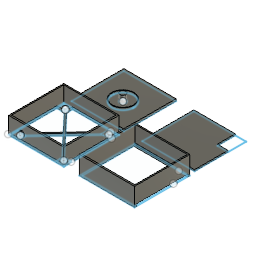
Enclosure_V2 (Autodesk Fusion 360 design; units mm, degrees)
part number: 2025-12-09-16-31-27-401
Autodesk Fusion 360 part; units mm, degrees
note: some values were not read from the file. Set by a fixed rule: which sketch regions a step uses.
sketch "Sketch1" plane through (0, 0, 0) normal (0, 0, 1) x (1, 0, 0)
  line L0 (19.5907, 74) -> (19.5907, 72.7904)
  line L1 (19.5907, 77.7937) -> (19.5907, 74)
  line L2 (78.8597, 77.7937) -> (71.7215, 77.7937)
  line L3 (44.546, 43.5668) -> (19.5907, 70.0195)
  line L4 (71.0242, 15.5) -> (46.0059, 42.0194)
  line L5 (78.8597, 70.2937) -> (78.8597, 77.7937)
  circle A0 centre (14.9411, 72.7904) radius 2.25
  circle A1 centre (73.9409, 72.7904) radius 2.25
  circle A2 centre (14.9411, 72.7904) radius 2.25
  line L6 (81.14, 79.55) -> (81.14, 4.55)
  line L7 (7.8597, 68.5) -> (7.8597, 77.7937)
  line L8 (71.0289, 68.5) -> (46.0059, 42.0194)
  line L9 (19.5907, 72.7904) -> (19.5907, 70.0195)
  circle A3 centre (14.9411, 72.7904) radius 2.25
  circle A4 centre (73.9409, 72.7904) radius 2.25
  line L10 (14, 68.5) -> (7.8597, 68.5)
  line L11 (18, 68.5) -> (14.9411, 68.5)
  line L12 (7.8597, 77.7937) -> (78.8597, 77.7937)
  line L13 (7.8597, 77.7937) -> (19.5907, 77.7937)
  line L14 (44.546, 43.5668) -> (68.0226, 68.411)
  line L15 (78.8597, 70.2937) -> (80.1709, 70.2937)
  line L16 (14, 68.5) -> (14.9411, 68.5)
  line L17 (6.14, 79.55) -> (81.14, 79.55)
  line L18 (6.14, 4.55) -> (6.14, 79.55)
  line L19 (7.8597, 6.7937) -> (7.8597, 77.7937)
  line L20 (78.8597, 77.7937) -> (78.8597, 6.7937)
  line L21 (78.8597, 15.5) -> (78.8597, 70.2937)
  line L22 (18, 68.5) -> (43.0327, 41.9653)
  circle A5 centre (14.9411, 11.728) radius 2.25
  line L23 (78.8597, 6.7937) -> (69.5, 6.7937)
  circle A6 centre (14.9411, 11.728) radius 2.25
  line L24 (14, 15.5) -> (7.8597, 15.5)
  circle A7 centre (73.9409, 11.728) radius 2.25
  line L25 (69.5, 6.7937) -> (69.5, 10.5)
  line L26 (19.5, 11.728) -> (19.5, 10.5)
  line L27 (44.4926, 40.4179) -> (69.5, 13.91)
  line L28 (81.14, 4.55) -> (6.14, 4.55)
  line L29 (69.5, 11.728) -> (69.5, 10.5)
  line L30 (7.8597, 6.7937) -> (19.5, 6.7937)
  line L31 (75, 15.5) -> (78.8597, 15.5)
  line L32 (69.5, 11.728) -> (69.5, 13.91)
  line L33 (19.5, 11.728) -> (19.5, 13.9695)
  line L34 (80.1709, 15.5) -> (78.8597, 15.5)
  line L35 (7.8597, 15.5) -> (7.8597, 6.7937)
  line L36 (44.4926, 40.4179) -> (19.5, 13.9695)
  line L37 (18.0242, 15.5) -> (43.0327, 41.9653)
  circle A8 centre (73.9409, 11.728) radius 2.25
  line L38 (19.5, 6.7937) -> (19.5, 10.5)
  line L39 (18.0242, 15.5) -> (14.9411, 15.5)
  line L40 (78.8597, 15.5) -> (78.8597, 6.7937)
  line L41 (71.0242, 15.5) -> (73.9409, 15.5)
  line L42 (73.9409, 15.5) -> (75, 15.5)
  line L43 (78.8597, 6.7937) -> (7.8597, 6.7937)
  line L44 (14, 15.5) -> (14.9411, 15.5)
  line L45 (71.0289, 68.5) -> (78.8597, 68.4104)
  line L46 (68.0226, 68.411) -> (68.0226, 77.7937)
  line L47 (81.14, 79.55) -> (81.14, 4.55)
  line L48 (81.14, 4.55) -> (6.14, 4.55)
  line L49 (6.14, 4.55) -> (6.14, 79.55)
  line L50 (6.14, 79.55) -> (81.14, 79.55)
  line L51 (177.14, 4.55) -> (102.14, 4.55)
  line L52 (102.14, 4.55) -> (102.14, 79.55)
  line L53 (102.14, 79.55) -> (177.14, 79.55)
  line L54 (177.14, 79.55) -> (177.14, 4.55)
  line L55 (104.3597, 77.7937) -> (175.3597, 77.7937)
  line L56 (175.3597, 77.7937) -> (175.3597, 6.7937)
  line L57 (175.3597, 6.7937) -> (104.3597, 6.7937)
  line L58 (104.3597, 6.7937) -> (104.3597, 77.7937)
  line L59 (175.3597, 77.7937) -> (164, 77.7937)
  line L60 (175.3597, 59) -> (175.3597, 77.7937)
  line L61 (104.3597, 157.7937) -> (175.3597, 157.7937)
  line L62 (175.3597, 157.7937) -> (175.3597, 87.7937)
  line L63 (104.3597, 87.7937) -> (104.3597, 157.7937)
  line L64 (175.3597, 87.7937) -> (104.3597, 87.7937)
  line L65 (80.3597, 86.7937) -> (9.3597, 86.7937)
  line L66 (9.3597, 157.7937) -> (80.3597, 157.7937)
  line L67 (80.3597, 157.7937) -> (80.3597, 86.7937)
  line L68 (9.3597, 86.7937) -> (9.3597, 157.7937)
  circle A9 centre (44.4231, 121.4369) radius 15
  line L69 (175.3597, 157.7937) -> (160.8017, 157.7937)
  line L70 (160.8017, 157.7937) -> (160.8017, 133.4306)
  line L71 (160.8017, 133.4306) -> (175.3597, 133.4306)
  line L72 (175.3597, 133.4306) -> (175.3597, 157.7937)
  circle A10 centre (44.4231, 121.4369) radius 14.2525
  line L73 (58.5254, 123.5) -> (59.2805, 123.5)
  line L74 (59.3541, 120) -> (58.6029, 120)
  line L75 (29.5408, 123.3128) -> (30.2946, 123.3128)
  line L76 (30.2432, 120) -> (29.492, 120)
  circle A11 centre (44.4231, 121.4369) radius 4.0094
  point P0 (5, 5)
  dimension "d1" = 4.5
  dimension "d2" = 4.5
  dimension "d3" = 4.5
  dimension "d4" = 4.5
  dimension "d5" = 7.5
  dimension "d7" = 4.5
  dimension "d8" = 4.5
  dimension "d9" = 4.5
  dimension "d10" = 4.5
  dimension "d11" = 4.5
  dimension "d12" = 75
  dimension "d13" = 75
  dimension "d14" = 71
  dimension "d15" = 71
  dimension "d17" = 75
  dimension "d18" = 75
  dimension "d19" = 75
  dimension "d20" = 75
  dimension "d21" = 71
  dimension "d36" = 70
  dimension "d41" = 71
  dimension "d42" = 30
  constraint horizontal L12
  constraint vertical L20
  constraint horizontal L43
  constraint vertical L19
  constraint horizontal L17
  constraint vertical L6
  constraint horizontal L28
  constraint vertical L18
  constraint horizontal L23
  constraint vertical L25
  constraint horizontal L41
  constraint vertical L40
  constraint horizontal L2
  constraint vertical L5
  constraint horizontal L13
  constraint vertical L1
  constraint horizontal L11
  constraint vertical L7
  constraint horizontal L30
  constraint vertical L38
  constraint horizontal L39
  constraint vertical L35
  constraint coincident L24.start L39
  constraint collinear L24 L39
  constraint coincident L26.start L38
  constraint collinear L33 L38
  constraint collinear L25 L32
  constraint coincident L31.start L41
  constraint collinear L31 L41
  constraint coincident L10.start L11
  constraint coincident L0.end L1
  constraint collinear L1 L9
  constraint collinear L10 L11
  constraint horizontal L15
  constraint horizontal L34
  constraint vertical L21
  constraint parallel L4 L22
  constraint parallel L8 L37
  constraint coincident L3.start L4
  constraint collinear L14 L37
  constraint collinear L3 L4
  constraint coincident L27.start L8
  constraint collinear L22 L27
  constraint collinear L8 L36
  constraint coincident L21 L45.end
  constraint coincident L12 L46.end
  constraint perpendicular L12 L46
  constraint horizontal L50
  constraint vertical L47
  constraint horizontal L48
  constraint vertical L49
  constraint horizontal L53
  constraint vertical L54
  constraint horizontal L51
  constraint vertical L52
  constraint horizontal L55
  constraint vertical L56
  constraint horizontal L57
  constraint vertical L58
  constraint horizontal L59
  constraint vertical L60
  constraint horizontal L61
  constraint vertical L62
  constraint horizontal L64
  constraint vertical L63
  constraint horizontal L66
  constraint vertical L67
  constraint horizontal L65
  constraint vertical L68
  constraint horizontal L69
  constraint vertical L70
  constraint horizontal L71
  constraint vertical L72
  constraint concentric A9 A10
  constraint horizontal L73
  constraint horizontal L74
  constraint coincident A10 L73.start
  constraint coincident A10 L74.end
  constraint coincident A9 L74.start
  constraint coincident A9 L73.end
  constraint horizontal L75
  constraint horizontal L76
  constraint coincident A9 L75.start
  constraint coincident A9 L76.end
  constraint coincident A10 L76.start
  constraint coincident A10 L75.end
  constraint concentric A9 A11
  measures "d1" diameter of A2
  measures "d2" diameter of A1
  measures "d3" diameter of A6
  measures "d4" diameter of A7
  measures "d5" distance of L2.start L5.start
  measures "d7" diameter of A0
  measures "d8" diameter of A4
  measures "d9" diameter of A5
  measures "d10" diameter of A8
  measures "d11" diameter of A3
  measures "d12" distance of L18.start L17.start
  measures "d13" distance of L6 L18
  measures "d14" distance of L19 L21
  measures "d15" distance of L12 L43
  measures "d17" distance of L18.start L17.start
  measures "d18" distance of L47 L49
  measures "d19" distance of L51.end L52.end
  measures "d20" distance of L52 L54
  measures "d21" distance of L55 L57
  measures "d36" distance of L61 L64
  measures "d41" distance of L65 L66
  measures "d42" diameter of A9
extrude "Extrude1" add sketch "Sketch1" along normal blind 3 contours L55 L56 L57 L58 L59 L60 makes body 1
extrude "Extrude2" add sketch "Sketch1" along normal blind 3 separate body contours L0 L1 L2 L3 L4 L5 L7 L8 L9 L10 L11 L12 L13 L14 L16 L19 L20 L21 L22 L23 L24 L25 L26 L27 L29 L30 L31 L32 L33 L35 L36 L37 L38 L39 L40 L41 L42 L43 L44 L45 L46 | L6 L17 L18 L28 L47 L48 L49 L50 makes body 2
extrude "Extrude3" add sketch "Sketch1" along normal blind 25 contours L51 L52 L53 L54 bodies 1
extrude "Extrude4" add sketch "Sketch1" along normal blind 23 separate body contours L6 L17 L18 L28 L47 L48 L49 L50 makes body 3
sketch "Sketch2" plane through (0, 4.55, 0) normal (0, -1, 0) x (1, 0, 0)
  line L0 (6.14, 0) -> (81.14, 0)
  line L1 (81.14, 0) -> (81.14, 23)
  line L2 (81.14, 23) -> (6.14, 23)
  line L3 (6.14, 23) -> (6.14, 0)
  line L4 (15, 15) -> (25, 15)
  line L5 (25, 15) -> (25, 5)
  line L6 (25, 5) -> (15, 5)
  line L7 (15, 5) -> (15, 15)
  constraint horizontal L4
  constraint vertical L5
  constraint horizontal L6
  constraint vertical L7
extrude "Extrude5" cut sketch "Sketch2" against normal blind 2 contours L4 L5 L6 L7 bodies 3
extrude "Extrude6" cut 1 faces at (18.3333, 6.55, 11.6667) along direction (0, 1, 0) blind 5 on bodies 3 bodies 3
extrude "Extrude7" cut 1 faces at (151.693, 30.4604, 3) along direction (0, 0, -1) blind 3 on bodies 1 bodies 1
extrude "Extrude8" add sketch "Sketch1" along normal blind 2 separate body contours L61 L62 L63 L64 L70 L71 | L61 L62 L69 L70 L71 L72 makes body 4
sketch "Sketch3" plane through (177.14, 0, 0) normal (1, 0, 0) x (0, 1, 0)
  line L0 (4.55, 0) -> (79.55, 0)
  line L1 (79.55, 0) -> (79.55, 25)
  line L2 (79.55, 25) -> (4.55, 25)
  line L3 (4.55, 25) -> (4.55, 0)
  line L4 (7, 3) -> (77.5, 3)
  line L5 (77.5, 3) -> (77.5, 1)
  line L6 (77.5, 1) -> (76, 0)
  line L7 (7, 3) -> (7, 1)
  line L8 (7, 1) -> (8.556, 0)
  constraint perpendicular L1 L4
  constraint perpendicular L0 L5
  constraint coincident L0 L6.end
  constraint perpendicular L4 L7
  constraint coincident L0 L8.end
extrude "Extrude9" cut sketch "Sketch3" against normal blind 3 contours L0 L4 L5 L6 L7 L8 bodies 1
extrude "Extrude10" add sketch "Sketch1" along normal blind 3 separate body contours L65 L66 L67 L68 makes body 5
sketch "Sketch4" plane through (175.3597, 0, 0) normal (-1, 0, 0) x (0, -1, 0)
  line L0 (-76, 0) -> (-77.5, 1)
  line L1 (-77.5, 1) -> (-77.5, 3)
  line L2 (-77.5, 3) -> (-7, 3)
  line L3 (-7, 3) -> (-7, 1)
  line L4 (-7, 1) -> (-8.556, 0)
  line L5 (-8.556, 0) -> (-6.7937, 0)
  line L6 (-6.7937, 0) -> (-6.7937, 25)
  line L7 (-6.7937, 25) -> (-77.7937, 25)
  line L8 (-77.7937, 25) -> (-77.7937, 0)
  line L9 (-77.7937, 0) -> (-76, 0)
  line L10 (-77.5, 3) -> (-77.7937, 3)
  line L11 (-7, 3) -> (-6.7937, 3)
  line L12 (-7, 3) -> (-7, 1)
  line L13 (-7, 1) -> (-8.556, 0)
  line L14 (-6.7937, 0) -> (-8.556, 0)
  line L15 (-6.7937, 3) -> (-6.7937, 0)
  constraint coincident L1.end L2.start
  constraint coincident L8 L10.end
  constraint perpendicular L8 L10
  constraint coincident L2.end L3.start
  constraint coincident L6 L11.end
  constraint perpendicular L6 L11
  constraint coincident L3.end L4.start
  constraint coincident L4.end L5.start
  constraint coincident L5.end L6.start
extrude "Extrude11" add sketch "Sketch4" along normal blind 71 contours L3 L4 L5 L6 L11 L12 L13 L14 L15 bodies 1
sketch "Sketch5" plane through (175.3597, 0, 0) normal (-1, 0, 0) x (0, -1, 0)
  line L0 (-7, 3) -> (-6.7937, 3)
  line L1 (-6.7937, 3) -> (-6.7937, 25)
  line L2 (-6.7937, 25) -> (-77.7937, 25)
  line L3 (-77.7937, 25) -> (-77.7937, 0)
  line L4 (-77.7937, 0) -> (-76, 0)
  line L5 (-76, 0) -> (-77.5, 1)
  line L6 (-77.5, 1) -> (-77.5, 3)
  line L7 (-77.5, 3) -> (-7, 3)
  line L8 (-77.5, 3) -> (-77.7937, 3)
  line L9 (-77.7937, 3) -> (-77.7937, 0)
  line L10 (-76, 0) -> (-77.5, 1)
  line L11 (-77.5, 3) -> (-77.5, 1)
  constraint coincident L6.end L7.start
  constraint coincident L3 L8.end
  constraint perpendicular L3 L8
  constraint coincident L3.end L4.start
  constraint coincident L4.end L5.start
  constraint coincident L5.end L6.start
extrude "Extrude12" add sketch "Sketch5" along normal blind 71 contours L3 L4 L5 L6 L8 L9 L10 L11 bodies 1
extrude "Extrude13" add sketch "Sketch1" along normal blind 2 separate body contours L61 L62 L63 L64 L70 L71 makes body 6
extrude "Extrude14" cut 1 faces at (151.693, 111.1271, 2) along direction (0, 0, -1) blind 3 on bodies 4 bodies 4 6
extrude "Extrude15" add sketch "Sketch1" along normal blind 2 contours L61 L62 L63 L64 L70 L71 bodies 4 6
extrude "Extrude16" add 1 faces at (18.3333, 6.0458, 5) along direction (0, 0, 1) blind 10 on bodies 3 bodies 3
sketch "Sketch6" plane through (0, 4.55, 0) normal (0, -1, 0) x (1, 0, 0)
  line L0 (6.14, 0) -> (81.14, 0)
  line L1 (81.14, 0) -> (81.14, 23)
  line L2 (81.14, 23) -> (6.14, 23)
  line L3 (6.14, 23) -> (6.14, 0)
  circle A0 centre (24.14, 10.2324) radius 3.7294
extrude "Extrude17" cut sketch "Sketch6" against normal blind 3 contours A0 bodies 3
extrude "Extrude18" add sketch "Sketch1" along normal blind 3 separate body contours A10 | A11 makes body 7
extrude "Extrude19" add sketch "Sketch1" along normal blind 2 separate body contours A9 A10 L73 L74 makes body 8
extrude "Extrude20" add sketch "Sketch1" along normal blind 2 separate body contours A9 A10 L75 L76 makes body 9
extrude "Extrude21" add sketch "Sketch1" along normal blind 10 separate body contours A11 makes body 10
